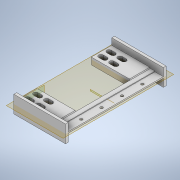
# Autodesk Inventor part: Rail_mount
Saved by Autodesk Inventor 2022 (Build 260153000, 153)
## iProperties
Created: 2021-07-29
Part Number: Rail_mount
Material: Generic
Document SubType Name: Modeling
Designer: exllu
Density: 1 g/cm^3
Appearance: Default
Mass: 2.05694 g
Surface Area: 45.935 cm^2
Volume: 2.05694 cm^3
Author: exllu
Autodesk Inventor part; units mm, degrees
ref_plane "YZ Plane" through (0, 0, 0) normal (1, 0, 0) x (0, 1, 0)
sketch "Sketch1" plane through (0, 0, 0) normal (0, 1, 0) x (-1, 0, 0)
  line L0 (0, 0) -> (-8, 0)
  line L1 (-8, 0) -> (-8, -70)
  line L2 (-8, -70) -> (0, -70)
  line L3 (0, -70) -> (0, 0)
  dimension "d0" = 8
  dimension "d1" = 70
  constraints: 8 end point, 2 parallel, 1 horizontal, 1 perpendicular
  measures "d0" distance of L2.end L1.end
  measures "d1" distance of L1.end L0.end
extrude "Extrusion1" add sketch "Sketch1" along normal blind 1
sketch "Sketch3" plane through (0, 0, 0) normal (0, -1, 0) x (1, 0, 0)
  line L0 (0, -70) -> (0, 0) projected
  line L1 (0, 0) -> (-10, 0)
  line L2 (-10, 0) -> (-10, -15)
  line L3 (-10, -15) -> (0, -15)
  line L4 (0, -15) -> (0, -35)
  line L5 (0, -70) -> (0, 0) projected
  line L6 (0, -35) -> (-8.8707, -35)
  line L7 (0, 0) -> (0, -70)
  line L8 (0, -70) -> (-10, -70)
  line L9 (-10, -70) -> (-10, -55)
  line L10 (-10, -55) -> (0, -55)
  dimension "d16" = 10
  dimension "d17" = 15
  dimension "d18" = 10
  constraints: 18 end point, 5 symmetric about line, 2 horizontal, 2 point on line, 1 midpoint, 1 perpendicular
  measures "d16" distance of L0.end L1.end
  measures "d17" distance of L1.end L2.end
  measures "d18" distance of L2.end L3.end
extrude "Extrusion3" add sketch "Sketch3" against normal blind 1
ref_plane "Work Plane1" through (8, 0, -35) normal (0, 0, 1) x (1, 0, 0)
sketch "Sketch4" plane through (8, 0, 0) normal (0, 0, 1) x (1, 0, 0)
  line L0 (0, 0) -> (0, 1) projected
  line L1 (0, 0) -> (0, -4.5)
  line L2 (0, -4.5) -> (-18, -4.5)
  line L3 (-18, -4.5) -> (-18, 0)
  line L4 (-18, 0) -> (-18, 1)
  line L5 (-18, 1) -> (-18, 5.5)
  line L6 (-18, 5.5) -> (0, 5.5)
  line L7 (0, 5.5) -> (0, 0)
  point P0 (-8, 0)
  dimension "d21" = 4.5
  dimension "d22" = 18
  dimension "d23" = 4.5
  dimension "d24" = 4.5
  dimension "d25" = 18
  constraints: 14 end point, 2 perpendicular, 2 point on line, 1 horizontal, 1 vertical
  measures "d21" distance of L0.start L1.end
  measures "d22" distance of L1.end L2.end
  measures "d23" distance of L2.end L3.end
  measures "d24" distance of L4.end L5.end
  measures "d25" distance of L5.end L6.end
extrude "Extrusion4" add sketch "Sketch4" along normal blind 1
mirror "Mirror1" about plane through (8, 0, -35) normal (0, 0, 1) of "Extrusion4"
sketch "Sketch5" plane through (0, 1, 0) normal (0, 1, 0) x (1, 0, 0)
  point P0 (0, 0)
sketch "Sketch6" plane through (0, 1, 0) normal (0, 1, 0) x (1, 0, 0)
  line L0 (-10, 0) -> (8, 0) projected
  line L1 (0, 0) -> (-10, 0)
  line L2 (-10, 0) -> (-10, 5)
  line L3 (-10, 15) -> (-10, 0) projected
  line L4 (-10, 5) -> (-10, 10)
  line L5 (-10, 10) -> (-7, 10)
  line L6 (-10, 5) -> (-7, 5)
  line L7 (-7, 5) -> (-4, 5)
  line L8 (-7, 10) -> (-5, 10)
  arc A0 (-7, 6.5) -> (-7, 3.5) centre (-7, 5) ccw
  arc A1 (-4, 3.5) -> (-4, 6.5) centre (-4, 5) ccw
  line L9 (-10, 7.5) -> (-7.9113, 7.5)
  line L10 (-7, 3.5) -> (-4, 3.5)
  line L11 (-7, 6.5) -> (-4, 6.5)
  dimension "d28" = 5
  dimension "d29" = 5
  dimension "d30" = 3
  dimension "d31" = 3
  dimension "d32" = 3
  dimension "d33" = 3
  dimension "d34" = 3
  constraints: 20 end point, 4 point on circle, 3 point on line, 2 centre point, 2 coincident, 2 horizontal, 2 perpendicular, 2 tangent, 1 collinear, 1 midpoint
  measures "d28" distance of L0.start L2.end
  measures "d29" distance of L2.end L4.end
  measures "d30" distance of L4.end L5.end
  measures "d31" distance of L2.end L6.end
  measures "d32" distance of L6.end L7.end
  measures "d33" diameter of A0
  measures "d34" diameter of A1
sketch "Sketch7" plane through (-10, 0, -15) normal (-1, 0, 0) x (0, 0, 1)
  line L0 (15, -4.5) -> (15, 0) projected
  line L1 (15, 0) -> (15, -4.5)
  line L2 (15, -4.5) -> (16, -4.5) projected
  line L3 (15, -4.5) -> (16, -4.5)
  line L4 (16, -4.5) -> (16, 5.5) projected
  line L5 (16, -4.5) -> (16, 5.5)
  line L6 (15, 5.5) -> (16, 5.5) projected
  line L7 (16, 5.5) -> (15, 5.5)
  line L8 (15, 1) -> (15, 5.5) projected
  line L9 (15, 5.5) -> (15, 1)
  line L10 (15, 1) -> (0, 1)
  line L11 (15, 1) -> (-55, 1) projected
  line L12 (0, 1) -> (0, 0)
  line L13 (15, 0) -> (0, 0) projected
  line L14 (0, 0) -> (15, 0)
  dimension "d35" = 15
  constraints: 16 end point, 4 collinear, 2 perpendicular, 1 point on line
  measures "d35" distance of L8.start L10.end
extrude "Extrusion5" add sketch "Sketch7" along normal blind 20
mirror "Mirror2" about plane through (8, 0, -35) normal (0, 0, 1) of "Extrusion5"
sketch "Sketch8" plane through (0, 1, 0) normal (0, 1, 0) x (1, 0, 0)
  line L0 (8, 0) -> (-30, 0) projected
  line L1 (0, 0) -> (-30, 0)
  line L2 (-30, 0) -> (-30, 5)
  line L3 (-30, 15) -> (-30, 0) projected
  line L4 (-30, 5) -> (-27, 5)
  line L5 (-27, 5) -> (-24, 5)
  arc A0 (-24, 3.375) -> (-24, 6.625) centre (-24, 5) ccw
  line L6 (-30, 5) -> (-30, 8)
  line L7 (-30, 8) -> (-28.0101, 8)
  line L8 (-27, 6.625) -> (-24, 6.625)
  line L9 (-27, 3.375) -> (-24, 3.375)
  arc A1 (-27, 6.625) -> (-27, 3.375) centre (-27, 5) ccw
  line L10 (-27, 11) -> (-24, 11)
  arc A2 (-24, 9.375) -> (-24, 12.625) centre (-24, 11) ccw
  line L11 (-27, 9.375) -> (-24, 9.375)
  line L12 (-27, 12.625) -> (-24, 12.625)
  arc A3 (-27, 12.625) -> (-27, 9.375) centre (-27, 11) ccw
  dimension "d38" = 5
  dimension "d39" = 3
  dimension "d40" = 3
  dimension "d42" = 3.25
  dimension "d43" = 3
  constraints: 22 end point, 8 point on circle, 8 symmetric about line, 4 centre point, 4 coincident, 3 point on line, 2 perpendicular, 2 tangent, 1 horizontal, 2 other
  measures "d38" distance of L0.end L2.end
  measures "d39" distance of L2.end L4.end
  measures "d40" distance of L4.end L5.end
  measures "d42" diameter of A0
  measures "d43" distance of L2.end L6.end
extrude "Extrusion6" cut sketch "Sketch8" against normal blind 4
mirror "Mirror3" about plane through (8, 0, -35) normal (0, 0, 1) of "Extrusion6"
sketch "Sketch9" plane through (0, 0, -55) normal (-1, 0, 0) x (0, 0, 1)
  line L0 (40, 0) -> (40, 1) projected
  line L1 (40, 1) -> (40.5, 1)
  line L2 (55, 1) -> (-15, 1) projected
  line L3 (40, 1) -> (40, 1.5)
  line L4 (40, 1.5) -> (0, 1.5)
  line L5 (0, 1.5) -> (0, -0.5)
  line L6 (0, -0.5) -> (40, -0.5)
  line L7 (40, -0.5) -> (40, 1.5)
  point P0 (55, 0)
  dimension "d46" = 0.5
  dimension "d47" = 0.5
  dimension "d48" = 40
  dimension "d49" = 2
  dimension "d50" = 40
  constraints: 12 end point, 2 vertical, 1 parallel, 1 perpendicular, 1 point on line
  measures "d46" distance of L0.end L1.end
  measures "d47" distance of L0.end L3.end
  measures "d48" distance of L3.end L4.end
  measures "d49" distance of L4.end L5.end
  measures "d50" distance of L5.end L6.end
ref_plane "Work Plane4" through (-21.5, 0, -15) normal (-1, 0, 0) x (0, 0, 1)
ref_plane "Work Plane3" through (-25.5, 0, -15) normal (-1, 0, 0) x (0, 0, 1)
mirror "Mirror4" about plane through (-21.5, 0, -15) normal (-1, 0, 0) of "Extrusion6", "Mirror3"
sketch "Sketch10" plane through (0, 1, 0) normal (0, 1, 0) x (1, 0, 0)
  line L0 (8, 0) -> (8, -1) projected
  line L1 (8, 0) -> (0, 0)
  line L2 (8, 0) -> (8, 70) projected
  line L3 (0, 0) -> (0, 12.5)
  line L4 (0, 12.5) -> (5, 12.5)
  line L5 (5, 12.5) -> (5, 27.5)
  circle A0 centre (5, 27.5) radius 1
  circle A1 centre (5, 12.5) radius 1
  point P0 (5, 13.5)
  point P1 (4, 12.5)
  dimension "d53" = 12.5
  dimension "d54" = 5
  dimension "d55" = 15
  dimension "d56" = 2
  dimension "d57" = 2
  constraints: 8 end point, 4 perpendicular, 2 centre point, 2 coincident
  measures "d53" distance of L1.end L3.end
  measures "d54" distance of L3.end L4.end
  measures "d55" distance of L4.end L5.end
  measures "d56" diameter of A0
  measures "d57" diameter of A1
extrude "Extrusion7" cut sketch "Sketch10" against normal blind 1
mirror "Mirror5" about plane through (8, 0, -35) normal (0, 0, 1) of "Extrusion7"
sketch "Sketch11" plane through (8, 0, 1) normal (0, 0, 1) x (1, 0, 0)
  line L0 (0, -4.5) -> (0, 0) projected
  line L1 (0, 1) -> (0, 5.5) projected
  line L2 (0, 0) -> (0, 5.5)
  line L3 (0, 5.5) -> (-38, 5.5) projected
  line L4 (0, -4.5) -> (-38, -4.5) projected
  line L5 (0, 5.5) -> (-38, 5.5)
  line L6 (-38, 5.5) -> (-38, -4.5)
  line L7 (-38, -4.5) -> (0, -4.5)
  line L8 (0, -4.5) -> (0, 5.5)
  point P0 (-8, 0)
  constraints: 10 end point, 2 parallel, 1 collinear, 1 horizontal, 1 perpendicular
extrude "Extrusion8" add sketch "Sketch11" along normal blind 1
mirror "Mirror6" about plane through (8, 0, -35) normal (0, 0, 1) of "Extrusion8"
sketch "Sketch12" plane through (8, 1, 0) normal (1, 0, 0) x (0, 0, -1)
  line L0 (0, -5.5) -> (0, -1) projected
  line L1 (0, -1) -> (0, -5)
  line L2 (0, -5) -> (0, -5.5)
  line L3 (0, -5.5) -> (-2, -5.5) projected
  line L4 (-2, -5.5) -> (-2, -5)
  line L5 (-2, 4.5) -> (-2, -5.5) projected
  line L6 (-2, -5) -> (0, -5)
  line L7 (0, -5) -> (0, -5.5)
  line L8 (0, -5.5) -> (-2, -5.5)
  line L9 (-2, -5.5) -> (-2, -5)
  line L10 (0, 0) -> (0, 4.5) projected
  line L11 (0, 4.5) -> (-2, 4.5)
  line L12 (-2, 4.5) -> (-2, 4)
  line L13 (-2, 4) -> (0, 4)
  line L14 (0, 4) -> (0, 4.5)
  point P0 (0, 4)
  dimension "d62" = 4
  dimension "d63" = 0.5
  constraints: 22 end point, 4 parallel, 3 point on line, 2 horizontal, 2 perpendicular, 1 collinear
  measures "d62" distance of L0.end L1.end
  measures "d63" distance of L12.end L11.end
extrude "Extrusion9" cut sketch "Sketch12" against normal blind 40
mirror "Mirror7" about plane through (8, 0, -35) normal (0, 0, 1) of "Extrusion9"
sketch "Sketch13" plane through (0, 1, 0) normal (0, 1, 0) x (1, 0, 0)
  line L0 (0, 15) -> (-30, 15) projected
  line L1 (-30, 0) -> (8, 0) projected
  line L2 (-30, 15) -> (-4, 15)
  line L3 (-4, 15) -> (-4, 0)
  line L4 (-4, 0) -> (-30, 0)
  line L5 (-30, 0) -> (-30, 15)
  arc A0 (-27, 6.625) -> (-27, 3.375) centre (-27, 5) ccw projected
  circle A1 centre (-27, 5) radius 1.55
  arc A2 (-27, 12.625) -> (-27, 9.375) centre (-27, 11) ccw projected
  circle A3 centre (-27, 11) radius 1.625
  arc A4 (-24, 9.375) -> (-24, 12.625) centre (-24, 11) ccw projected
  circle A5 centre (-24, 11) radius 1.625
  arc A6 (-24, 3.375) -> (-24, 6.625) centre (-24, 5) ccw projected
  circle A7 centre (-24, 5) radius 1.625
  arc A8 (-19, 6.625) -> (-19, 3.375) centre (-19, 5) ccw projected
  circle A9 centre (-19, 5) radius 1.625
  arc A10 (-19, 12.625) -> (-19, 9.375) centre (-19, 11) ccw projected
  circle A11 centre (-19, 11) radius 1.55
  arc A12 (-16, 9.375) -> (-16, 12.625) centre (-16, 11) ccw projected
  circle A13 centre (-16, 11) radius 1.625
  arc A14 (-16, 3.375) -> (-16, 6.625) centre (-16, 5) ccw projected
  circle A15 centre (-16, 5) radius 1.625
  line L6 (-27, 6.625) -> (-24, 6.625) projected
  line L7 (-27, 6.625) -> (-24, 6.625)
  line L8 (-24, 3.375) -> (-27, 3.375) projected
  line L9 (-27, 3.375) -> (-24, 3.375)
  line L10 (-27, 12.625) -> (-24, 12.625) projected
  line L11 (-27, 12.625) -> (-24, 12.625)
  line L12 (-27, 9.375) -> (-24, 9.375) projected
  line L13 (-27, 9.375) -> (-24, 9.375)
  line L14 (-16, 12.625) -> (-19, 12.625) projected
  line L15 (-19, 12.625) -> (-16, 12.625)
  line L16 (-16, 9.375) -> (-19, 9.375) projected
  line L17 (-19, 9.375) -> (-16, 9.375)
  line L18 (-16, 6.625) -> (-19, 6.625) projected
  line L19 (-19, 6.625) -> (-16, 6.625)
  line L20 (-19, 3.375) -> (-16, 3.375) projected
  line L21 (-19, 3.375) -> (-16, 3.375)
  point P0 (0, 0)
  dimension "d66" = 26
  constraints: 24 end point, 9 equal length, 8 coincident, 7 tangent, 6 centre point, 4 horizontal, 3 point on line, 2 vertical alignment, 1 perpendicular, 4 other
  measures "d66" distance of L3.end L4.end
extrude "Extrusion10" add sketch "Sketch13" along normal blind 3
mirror "Mirror8" about plane through (8, 0, -35) normal (0, 0, 1) of "Extrusion10"
chamfer "Chamfer1" distance 3 angle 45 2 edges at (-4, 1, -7.5) (-4, 1, -62.5)
ref_plane "Work Plane5" through (0, 0.5, 0) normal (0, 1, 0) x (1, 0, 0)
mirror "Mirror9" about plane through (0, 0.5, 0) normal (0, 1, 0) of "Extrusion10"
mirror "Mirror10" about plane through (0, 0.5, 0) normal (0, 1, 0) of "Extrusion10", "Mirror8"
chamfer "Chamfer2" distance 3 angle 45 2 edges at (-4, 0, -7.5) (-4, 0, -62.5)
sketch "Sketch14" plane through (0, 4, 0) normal (0, 1, 0) x (1, 0, 0)
  line L0 (0, 0) -> (-43.4842, 0)
  line L1 (-43.4842, 0) -> (-43.4842, 70)
  line L2 (-43.4842, 70) -> (0, 70)
  line L3 (0, 70) -> (0, 0)
  constraints: 8 end point, 2 parallel, 1 horizontal, 1 perpendicular
extrude "Extrusion11" cut sketch "Sketch14" against normal blind 2
sketch "Sketch15" plane through (0, 1, 0) normal (0, 1, 0) x (1, 0, 0)
  line L0 (8, 0) -> (8, 70) projected
  line L1 (8, 0) -> (1.8, 0)
  line L2 (-1, 0) -> (8, 0) projected
  line L3 (1.8, 0) -> (1.8, 70)
  line L4 (-30, 70) -> (8, 70) projected
  line L5 (8, 72) -> (8, 70) projected
  line L6 (8, 70) -> (1.8, 70)
  line L7 (1.8, 0) -> (-1.5, 0)
  line L8 (-1.5, 0) -> (-1.5, 70)
  line L9 (-1.5, 70) -> (1.8, 70)
  line L10 (1.8, 70) -> (1.8, 0)
  point P0 (0, 0)
  dimension "d78" = 6.2
  dimension "d79" = 3.3
  constraints: 14 end point, 3 perpendicular, 3 point on line, 2 parallel, 1 horizontal
  measures "d78" distance of L0.start L1.end
  measures "d79" distance of L8.end L9.end
extrude "Extrusion12" add sketch "Sketch15" along normal mid plane 1 contours L2 L7 L8 L4 L3
mirror "Mirror11" about plane through (0, 0.5, 0) normal (0, 1, 0) of "Extrusion12"
sketch "Sketch16" plane through (-30, -4, -72) normal (0, -1, 0) x (1, 0, 0)
  line L0 (38, 0) -> (0, 0) projected
  line L1 (0, 0) -> (38, 0)
  line L2 (38, 0) -> (38, 2)
  line L3 (38, 2) -> (0, 2)
  line L4 (0, 2) -> (0, 0)
  line L5 (38, 74) -> (0, 74) projected
  line L6 (0, 72) -> (38, 72) projected
  line L7 (0, 74) -> (38, 74)
  line L8 (38, 74) -> (38, 72)
  line L9 (38, 72) -> (0, 72)
  line L10 (0, 72) -> (0, 74)
  point P0 (30, 72)
  constraints: 16 end point, 4 parallel, 2 horizontal, 2 perpendicular
extrude "Extrusion13" add sketch "Sketch16" along normal blind 1.8
mirror "Mirror12" about plane through (0, 0.5, 0) normal (0, 1, 0) of "Extrusion13"
ref_plane "Work Plane2" through (8, 0, -35) normal (0, 0, 1) x (1, 0, 0)
body "Solid1"
